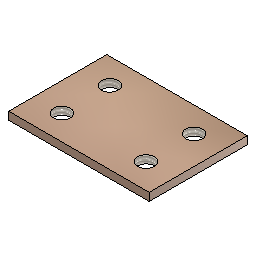
Copper Busbar - Series Link v4 (Autodesk Fusion 360 design; units mm, degrees)
Autodesk Fusion 360 part; units mm, degrees
sketch "Sketch1" plane through (0, 0, 0) normal (0, 1, 0) x (1, 0, 0)
  line L0 (0, 0) -> (28.65, 0)
  line L1 (28.65, 0) -> (28.65, 20)
  line L2 (28.65, 20) -> (0, 20)
  line L3 (0, 20) -> (0, 0)
  circle A0 centre (5.75, 14.89) radius 1.727
  circle A1 centre (5.75, 5.11) radius 1.727
  line L4 (14.325, 20) -> (14.325, 0) construction
  circle A2 centre (22.9, 14.89) radius 1.727
  circle A3 centre (22.9, 5.11) radius 1.727
  dimension "d1" = 20
  dimension "d2" = 28.65
  dimension "d3" = 3.454
  dimension "d4" = 3.454
  dimension "d5" = 5.11
  dimension "d6" = 9.78
  dimension "d7" = 5.237
  dimension "d8" = 5.75
  dimension "d9" = 14.325
  dimension "d10" = 5.75
  dimension "d13" = 16
  constraint horizontal L0
  constraint vertical L1
  constraint horizontal L2
  constraint vertical L3
  constraint coincident L0.start L3.end
  constraint vertical A0.centre A1.centre
  constraint coincident L0 L4.end
  constraint perpendicular L0 L4
  constraint symmetric A0 L4 A2
  constraint symmetric A1 L4 A3
  measures "d1" distance of L0.start L2.end
  measures "d2" distance of L1.end L2.end
  measures "d3" diameter of A0
  measures "d4" diameter of A1
  measures "d5" distance of L2 A0.centre
  measures "d6" distance of A0.centre A1.centre
  measures "d8" horizontal distance of L2.end A0.centre
  measures "d9" distance of L0.start L4
  measures "d10" horizontal distance of L1.end A2.centre
extrude "Extrude1" add sketch "Sketch1" along normal blind 1.6
thread "Thread1" "ANSI Unified Screw Threads 0.164(#8) 8-32 UNC 3B" major diameter 4.1656 minor diameter 3.4163 pitch 0.7937 angle 60 resizes the face on face at (7.4684, 1.0667, -14.718) on face at (24.6184, 1.0667, -14.718) on face at (24.6184, 1.0667, -4.938) on face at (7.4684, 1.0667, -4.938)
equation "d9 = ( 28.65 / 2 ) * 1 mm"
